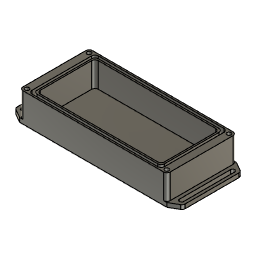
Universal case (Autodesk Fusion 360 design; units mm, degrees)
Autodesk Fusion 360 part; units mm, degrees
sketch "Sketch1" plane through (0, 0, 0) normal (0, 0, 1) x (1, 0, 0)
  line L0 (37.5, 17.5) -> (-37.5, 17.5)
  line L1 (-37.5, 17.5) -> (-37.5, -17.5)
  line L2 (-37.5, -17.5) -> (37.5, -17.5)
  line L3 (37.5, -17.5) -> (37.5, 17.5)
  line L4 (37.5, 17.5) -> (-37.5, -17.5) construction
  line L5 (-37.5, 17.5) -> (37.5, -17.5) construction
  line L6 (44.5, 21) -> (-44.5, 21)
  line L7 (-44.5, 21) -> (-44.5, -21)
  line L8 (-44.5, -21) -> (44.5, -21)
  line L9 (44.5, -21) -> (44.5, 21)
  line L10 (44.5, 21) -> (-44.5, -21) construction
  line L11 (-44.5, 21) -> (44.5, -21) construction
  line L12 (0, 2.5) -> (0, 20)
  line L13 (44.5, -21) -> (50.75, -17.3916)
  line L14 (50.75, -17.3916) -> (50.75, 17.3916)
  line L15 (50.75, 17.3916) -> (44.5, 21)
  line L16 (46.5, 15.5) -> (46.5, -15.5)
  arc A0 (46.5, -15.5) -> (49, -15.5) centre (47.75, -15.5) ccw
  line L17 (49, -15.5) -> (49, 15.5)
  arc A1 (49, 15.5) -> (46.5, 15.5) centre (47.75, 15.5) ccw
  line L18 (47.75, 15.5) -> (47.75, -15.5) construction
  arc A2 (-49, -15.5) -> (-46.5, -15.5) centre (-47.75, -15.5) ccw
  line L19 (-46.5, 15.5) -> (-46.5, -15.5)
  line L20 (-49, -15.5) -> (-49, 15.5)
  arc A3 (-46.5, 15.5) -> (-49, 15.5) centre (-47.75, 15.5) ccw
  line L21 (-50.75, 17.3916) -> (-44.5, 21)
  line L22 (-50.75, -17.3916) -> (-50.75, 17.3916)
  line L23 (-44.5, -21) -> (-50.75, -17.3916)
  line L24 (38.5, 18.5) -> (-38.5, 18.5)
  line L25 (-38.5, 18.5) -> (-38.5, -18.5)
  line L26 (-38.5, -18.5) -> (38.5, -18.5)
  line L27 (38.5, -18.5) -> (38.5, 18.5)
  line L28 (38.5, 18.5) -> (-38.5, -18.5) construction
  line L29 (-38.5, 18.5) -> (38.5, -18.5) construction
  line L30 (40, 20) -> (-40, 20)
  line L31 (-40, 20) -> (-40, -20)
  line L32 (-40, -20) -> (40, -20)
  line L33 (40, -20) -> (40, 20)
  line L34 (40, 20) -> (-40, -20) construction
  line L35 (-40, 20) -> (40, -20) construction
  circle A4 centre (42.25, 18.75) radius 1.25
  circle A5 centre (-42.25, 18.75) radius 1.25
  line L36 (20, 0) -> (2.5, 0)
  circle A6 centre (42.25, -18.75) radius 1.25
  circle A7 centre (-42.25, -18.75) radius 1.25
  line L37 (-107, 0) -> (107, 0)
  point P0 (47.75, 0)
  dimension "d1" = 35
  dimension "d3" = 75
  dimension "d26" = 120
  dimension "d46" = 3.5
  dimension "d47" = 1
  dimension "d48" = 1
  dimension "d49" = 1
  dimension "d51" = 1.5
  dimension "d52" = 89
  dimension "d53" = 2.5
  dimension "d54" = 2.25
  dimension "d55" = 2.25
  dimension "d56" = 2.5
  dimension "d57" = 6.25
  dimension "d66" = 2
  dimension "d67" = 31
  constraint horizontal L0
  constraint perpendicular L0 L1
  constraint parallel L0 L2
  constraint parallel L1 L3
  constraint coincident L4 origin
  constraint coincident L5 origin
  constraint horizontal L6
  constraint perpendicular L6 L7
  constraint parallel L6 L8
  constraint parallel L7 L9
  constraint coincident L10 origin
  constraint coincident L11 origin
  constraint perpendicular L8 L14
  constraint tangent L16 A0
  constraint tangent A0 L17
  constraint parallel L16 L17
  constraint tangent L17 A1
  constraint tangent L16 A1
  constraint parallel L9 L18
  constraint symmetric L6.start L12 L6.end
  constraint symmetric L8.end L12 L7.end
  constraint symmetric L12 L13.end L22.start
  constraint symmetric L12 L14.end L21.start
  constraint symmetric L12 L16.start L19.start
  constraint symmetric L12 L16.end A2.end
  constraint symmetric L12 A0.end A2.start
  constraint symmetric L12 L17.end L20.end
  constraint symmetric L12 A0 A2
  constraint symmetric L12 A1 A3
  constraint horizontal L24
  constraint perpendicular L24 L25
  constraint parallel L24 L26
  constraint parallel L25 L27
  constraint coincident L28 origin
  constraint coincident L29 origin
  constraint horizontal L30
  constraint perpendicular L30 L31
  constraint parallel L30 L32
  constraint parallel L31 L33
  constraint coincident L34 origin
  constraint coincident L35 origin
  constraint symmetric L12 A4 A5
  constraint symmetric A4 L36 A6
  constraint symmetric A5 L36 A7
  constraint horizontal L37
  constraint midpoint L37 origin
  constraint midpoint L18 P0
  constraint coincident L37 P0
  constraint equal L13 L15
  measures "d1" distance of L0.start L2.end
  measures "d3" distance of L0.start L0.end
  measures "d26" angle of L13 L14
  measures "d46" distance of L0 L6
  measures "d47" distance of L0 L24
  measures "d48" distance of L6 L30
  measures "d49" distance of L1 L25
  measures "d51" distance of L25 L31
  measures "d52" distance of L6.start L6.end
  measures "d53" diameter of A4
  measures "d54" distance of L6 A4.centre
  measures "d55" distance of L9 A4.centre
  measures "d56" distance of L16 L17
  measures "d57" distance of L9 L14
  measures "d66" distance of L9 L16
  measures "d67" distance of A1.centre A0.centre
extrude "Extrude2" add sketch "Sketch1" along normal blind 2.5 contours L0 L1 L3 L36 L37 | L0 L3 L12 L24 L27 L37 | L0 L1 L12 L24 L25 L37 | L1 L2 L3 L25 L26 L27 L37 | L1 L2 L3 L36 L37 | L12 L24 L25 L30 L31 L37 | L12 L24 L27 L30 L33 L37 | L25 L26 L27 L31 L32 L33 L37 | L6 L7 L9 L30 L31 L33 L37 | L7 L8 L9 L31 L32 L33 L37 | L9 L13 L14 L16 A0 L17 L37 | L9 L14 L15 L16 L17 A1 L37 | L7 L19 L20 A3 L21 L22 L37 | L7 A2 L19 L20 L22 L23 L37
extrude "Extrude14" add sketch "Sketch1" along normal blind 15 from surface at 2.5 contours L0 L3 L12 L24 L27 L37 | L0 L1 L12 L24 L25 L37 | L1 L2 L3 L25 L26 L27 L37 | L12 L24 L25 L30 L31 L37 | L12 L24 L27 L30 L33 L37 | L25 L26 L27 L31 L32 L33 L37 | L6 L7 L9 L30 L31 L33 L37 | L7 L8 L9 L31 L32 L33 L37 | A4 | A5 | A6 | A7
extrude "Extrude15" cut sketch "Sketch1" against normal blind 5 from surface at 17.5 contours L12 L24 L25 L30 L31 L37 | L12 L24 L27 L30 L33 L37 | L25 L26 L27 L31 L32 L33 L37
extrude "Extrude16" cut sketch "Sketch1" against normal blind 10 from surface at 17.5 contours A4 | A5 | A6 | A7
fillet "Fillet5" radius 2 20 edges at (-50.75, -17.3916, 1.25) (-44.5, -21, 10) (-50.75, 17.3916, 1.25) (-44.5, 21, 10) (-38.5, 18.5, 15) (-40, 20, 15) (-37.5, 17.5, 10) (-37.5, -17.5, 10) (-38.5, -18.5, 15) (-40, -20, 15) (37.5, 17.5, 10) (40, 20, 15) (37.5, -17.5, 10) (38.5, -18.5, 15) (40, -20, 15) (44.5, -21, 10) (50.75, -17.3916, 1.25) (38.5, 18.5, 15) (44.5, 21, 10) (50.75, 17.3916, 1.25)
equation "d7 = 2.50 mm"
equation "d48 = d47"
equation "d49 = d47"
equation "d51 = d46 - 2 * d47"
equation "d52 = d3 + 2 * d46 + 2 * d47 + 2 * d53"
equation "d54 = d47 + 0.5 * d53"
equation "d55 = d47 + 0.5 * d53"
equation "d56 = d53"
equation "d57 = d54 + 4 * d47"
equation "d66 = 2 * d47"
equation "d67 = d1 - 4 * d47"
equation "d80 = d7"
equation "d81 = 15 mm"
equation "d83 = d7 + d81"
equation "d86 = d7 + d81"
